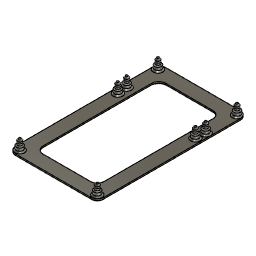
ESPBoardWithSenseHATHolder (Autodesk Fusion 360 design; units mm, degrees)
Autodesk Fusion 360 part; units mm, degrees
note: some values were not read from the file. Set by a fixed rule: which face or edge a step refers to.
sketch "Sketch1" plane through (0, 0, 0) normal (0, 0, 1) x (1, 0, 0)
  line L0 (27.5, -55) -> (-27.5, -55)
  line L1 (-32.5, -50) -> (-32.5, 50)
  line L2 (-27.5, 55) -> (27.5, 55)
  line L3 (32.5, 50) -> (32.5, -50)
  line L4 (32.5, -55) -> (-32.5, 55) construction
  line L5 (-32.5, -55) -> (32.5, 55) construction
  circle A0 centre (28.45, -51) radius 1.5
  circle A1 centre (28.45, 21) radius 1.5
  line L6 (28.45, -51) -> (28.45, 23.226) construction
  circle A2 centre (29, 28) radius 1.5
  line L7 (29, 28) -> (29, 54) construction
  circle A3 centre (29, 51) radius 1.5
  circle A4 centre (28.45, -51) radius 2.1
  circle A5 centre (28.45, 21) radius 2.1
  circle A6 centre (29, 28) radius 2.1
  circle A7 centre (29, 51) radius 2.1
  line L8 (29.3, 48.9) -> (28.7, 48.9)
  line L9 (28.7, 48.9) -> (28.7, 53.1)
  line L10 (28.7, 53.1) -> (29.3, 53.1)
  line L11 (29.3, 53.1) -> (29.3, 48.9)
  line L12 (29.3, 48.9) -> (28.7, 53.1) construction
  line L13 (28.7, 48.9) -> (29.3, 53.1) construction
  line L14 (29.3, 25.9) -> (28.7, 25.9)
  line L15 (28.7, 25.9) -> (28.7, 30.1)
  line L16 (28.7, 30.1) -> (29.3, 30.1)
  line L17 (29.3, 30.1) -> (29.3, 25.9)
  line L18 (29.3, 25.9) -> (28.7, 30.1) construction
  line L19 (28.7, 25.9) -> (29.3, 30.1) construction
  line L20 (28.75, 18.9) -> (28.15, 18.9)
  line L21 (28.15, 18.9) -> (28.15, 23.1)
  line L22 (28.15, 23.1) -> (28.75, 23.1)
  line L23 (28.75, 23.1) -> (28.75, 18.9)
  line L24 (28.75, 18.9) -> (28.15, 23.1) construction
  line L25 (28.15, 18.9) -> (28.75, 23.1) construction
  line L26 (28.75, -53.1) -> (28.15, -53.1)
  line L27 (28.15, -53.1) -> (28.15, -48.9)
  line L28 (28.15, -48.9) -> (28.75, -48.9)
  line L29 (28.75, -48.9) -> (28.75, -53.1)
  line L30 (28.75, -53.1) -> (28.15, -48.9) construction
  line L31 (28.15, -53.1) -> (28.75, -48.9) construction
  line L32 (0, 55) -> (0, -55) construction
  circle A8 centre (-29, 28) radius 2.1
  line L33 (-29.3, 30.1) -> (-29.3, 25.9)
  line L34 (-28.7, 48.9) -> (-28.7, 53.1)
  circle A9 centre (-28.45, 21) radius 2.1
  line L35 (-29.3, 48.9) -> (-28.7, 48.9)
  line L36 (-28.7, 48.9) -> (-29.3, 53.1) construction
  line L37 (-28.15, -53.1) -> (-28.75, -48.9) construction
  line L38 (-28.75, -53.1) -> (-28.15, -53.1)
  circle A10 centre (-28.45, 21) radius 1.5
  circle A11 centre (-28.45, -51) radius 1.5
  line L39 (-28.15, -53.1) -> (-28.15, -48.9)
  line L40 (-28.7, 25.9) -> (-29.3, 30.1) construction
  line L41 (-28.15, -48.9) -> (-28.75, -48.9)
  line L42 (-28.75, -48.9) -> (-28.75, -53.1)
  line L43 (-28.75, 18.9) -> (-28.15, 18.9)
  line L44 (-28.75, -53.1) -> (-28.15, -48.9) construction
  circle A12 centre (-28.45, -51) radius 2.1
  line L45 (-28.15, 18.9) -> (-28.75, 23.1) construction
  circle A13 centre (-29, 51) radius 2.1
  line L46 (-29.3, 53.1) -> (-29.3, 48.9)
  circle A14 centre (-29, 51) radius 1.5
  line L47 (-28.15, 18.9) -> (-28.15, 23.1)
  line L48 (-28.7, 30.1) -> (-29.3, 30.1)
  circle A15 centre (-29, 28) radius 1.5
  line L49 (-29.3, 25.9) -> (-28.7, 25.9)
  line L50 (-29.3, 48.9) -> (-28.7, 53.1) construction
  line L51 (-28.7, 25.9) -> (-28.7, 30.1)
  line L52 (-28.75, 23.1) -> (-28.75, 18.9)
  line L53 (-28.15, 23.1) -> (-28.75, 23.1)
  line L54 (-28.7, 53.1) -> (-29.3, 53.1)
  line L55 (-29.3, 25.9) -> (-28.7, 30.1) construction
  line L56 (-28.75, 18.9) -> (-28.15, 23.1) construction
  line L57 (17.5, -45) -> (-17.5, -45)
  line L58 (-22.5, -40) -> (-22.5, 40)
  line L59 (-17.5, 45) -> (17.5, 45)
  line L60 (22.5, 40) -> (22.5, -40)
  arc A16 (-17.5, 45) -> (-22.5, 40) centre (-17.5, 40) ccw
  arc A17 (-27.5, 55) -> (-32.5, 50) centre (-27.5, 50) ccw
  arc A18 (32.5, 50) -> (27.5, 55) centre (27.5, 50) ccw
  arc A19 (27.5, -55) -> (32.5, -50) centre (27.5, -50) ccw
  arc A20 (-32.5, -50) -> (-27.5, -55) centre (-27.5, -50) ccw
  arc A21 (-22.5, -40) -> (-17.5, -45) centre (-17.5, -40) ccw
  arc A22 (17.5, -45) -> (22.5, -40) centre (17.5, -40) ccw
  arc A23 (22.5, 40) -> (17.5, 45) centre (17.5, 40) ccw
  circle A24 centre (28.45, -51) radius 2.5
  circle A25 centre (28.45, 21) radius 2.5
  circle A26 centre (29, 28) radius 2.5
  circle A27 centre (29, 51) radius 2.5
  circle A28 centre (-29, 51) radius 2.5
  circle A29 centre (-29, 28) radius 2.5
  circle A30 centre (-28.45, 21) radius 2.5
  circle A31 centre (-28.45, -51) radius 2.5
  point P0 (29, 51)
  point P1 (29, 28)
  point P2 (28.45, 21)
  point P3 (28.45, -51)
  point P4 (-28.45, 23.226)
  point P5 (-28.45, 21)
  point P6 (-29, 28)
  point P7 (-29, 51)
  point P8 (-28.45, -51)
  point P9 (-28.45, -51)
  point P10 (-29, 28)
  dimension "d1" = 65
  dimension "d2" = 110
  dimension "d5" = 3
  dimension "d6" = 4.05
  dimension "d7" = 4
  dimension "d8" = 3
  dimension "d9" = 72
  dimension "d10" = 3
  dimension "d11" = 7
  dimension "d12" = 0.55
  dimension "d13" = 3
  dimension "d14" = 23
  dimension "d15" = 4.2
  dimension "d16" = 4.2
  dimension "d17" = 4.2
  dimension "d18" = 4.2
  dimension "d19" = 0.6
  dimension "d20" = 4.2
  dimension "d21" = 0.6
  dimension "d22" = 4.2
  dimension "d23" = 0.6
  dimension "d24" = 4.2
  dimension "d25" = 0.6
  dimension "d26" = 4.2
  dimension "d28" = 5
  dimension "d43" = 56.9
  dimension "d44" = 58
  dimension "d49" = 5
  dimension "d50" = 5
  dimension "d51" = 5
  dimension "d52" = 5
  constraint horizontal L0
  constraint perpendicular L0 L1
  constraint parallel L0 L2
  constraint parallel L1 L3
  constraint coincident L4 origin
  constraint coincident L5 origin
  constraint coincident P3 A0.centre
  constraint parallel L3 L6
  constraint coincident P2 L6
  constraint coincident P1 A2.centre
  constraint vertical L7
  constraint coincident L7 P0
  constraint concentric A0 A4
  constraint concentric A1 A5
  constraint concentric A2 A6
  constraint concentric A3 A7
  constraint horizontal L8
  constraint perpendicular L8 L9
  constraint parallel L8 L10
  constraint parallel L9 L11
  constraint coincident L12 P0
  constraint coincident L13 P0
  constraint coincident P0 A3.centre
  constraint horizontal L14
  constraint perpendicular L14 L15
  constraint parallel L14 L16
  constraint parallel L15 L17
  constraint coincident L18 P1
  constraint coincident L19 P1
  constraint horizontal L20
  constraint perpendicular L20 L21
  constraint parallel L20 L22
  constraint parallel L21 L23
  constraint coincident L24 P2
  constraint coincident L25 P2
  constraint coincident P2 A1.centre
  constraint horizontal L26
  constraint perpendicular L26 L27
  constraint parallel L26 L28
  constraint parallel L27 L29
  constraint coincident L30 P3
  constraint coincident L31 P3
  constraint symmetric A0 L32 A11
  constraint symmetric A1 L32 A10
  constraint symmetric P3 L32 P9
  constraint symmetric L6.end L32 P4
  constraint symmetric A2 L32 A15
  constraint symmetric P1 L32 P10
  constraint symmetric A3 L32 A14
  constraint symmetric A4 L32 A12
  constraint symmetric A5 L32 A9
  constraint symmetric A6 L32 A8
  constraint symmetric A7 L32 A13
  constraint symmetric L8.start L32 L35.start
  constraint symmetric L8.end L32 L34.start
  constraint symmetric L9.end L32 L34.end
  constraint symmetric L10.end L32 L36.end
  constraint symmetric P0 L32 P7
  constraint symmetric L14.start L32 L33.end
  constraint symmetric L14.end L32 L40.start
  constraint symmetric L15.end L32 L48.start
  constraint symmetric L16.end L32 L33.start
  constraint symmetric L20.start L32 L43.start
  constraint symmetric L20.end L32 L43.end
  constraint symmetric L21.end L32 L47.end
  constraint symmetric L22.end L32 L45.end
  constraint symmetric P2 L32 P5
  constraint symmetric L26.start L32 L38.start
  constraint symmetric L26.end L32 L37.start
  constraint symmetric L27.end L32 L39.end
  constraint symmetric L28.end L32 L37.end
  constraint tangent L58 A16
  constraint tangent L59 A16
  constraint coincident L2 L32.start
  constraint coincident L4.end L1
  constraint coincident L4.end L2
  constraint tangent L1 A17
  constraint tangent L2 A17
  constraint equal A16 A17
  constraint coincident L5.end L2
  constraint coincident L5.end L3
  constraint tangent L2 A18
  constraint tangent L3 A18
  constraint equal A16 A18
  constraint coincident L0 L32.end
  constraint coincident L4.start L3
  constraint coincident L4.start L0
  constraint tangent L3 A19
  constraint tangent L0 A19
  constraint equal A16 A19
  constraint coincident L5.start L0
  constraint coincident L5.start L1
  constraint tangent L0 A20
  constraint tangent L1 A20
  constraint equal A16 A20
  constraint tangent L57 A21
  constraint tangent L58 A21
  constraint equal A16 A21
  constraint tangent L60 A22
  constraint tangent L57 A22
  constraint equal A16 A22
  constraint tangent L60 A23
  constraint tangent L59 A23
  constraint equal A16 A23
  constraint concentric A5 A25
  constraint concentric A6 A26
  constraint concentric A7 A27
  constraint symmetric L32 A24 A31
  constraint symmetric L32 A25 A30
  constraint symmetric L32 A26 A29
  constraint symmetric L32 A27 A28
  measures "d1" distance of L4.end L5.end
  measures "d2" distance of L5.start L4.end
  measures "d5" diameter of A0
  measures "d6" distance of L3 P3
  measures "d7" distance of L0 P3
  measures "d8" diameter of A1
  measures "d9" vertical distance of P3 P2
  measures "d10" diameter of A2
  measures "d11" vertical distance of P2 P1
  measures "d12" distance of L6 P1
  measures "d13" diameter of A3
  measures "d14" distance of P1 P0
  measures "d15" diameter of A4
  measures "d16" diameter of A5
  measures "d17" diameter of A6
  measures "d18" diameter of A7
  measures "d19" distance of L9.end L10.end
  measures "d20" distance of L8.end L9.end
  measures "d21" distance of L15.end L16.end
  measures "d22" distance of L14.end L15.end
  measures "d23" distance of L21.end L22.end
  measures "d24" distance of L20.end L21.end
  measures "d25" distance of L27.end L28.end
  measures "d26" distance of L26.end L27.end
  measures "d28" radius of A16 L11
  measures "d43" distance of P3 P9
  measures "d44" distance of P0 P7
  measures "d49" diameter of A24
  measures "d50" diameter of A25
  measures "d51" diameter of A26
  measures "d52" diameter of A27
extrude "Extrude1" add sketch "Sketch1" against normal blind 2 contours L0 L1 L2 L3 A17 A18 A19 A20 | A0 L29 | A0 A4 L29 | A0 L27 L29 | A0 A4 L27 L29 | A0 A4 L27 L29 | A0 L27 | A0 A4 L27 | A4 L28 L29 | A4 L26 L29 | A4 L27 L28 | A4 L26 L27 | A1 L23 | A1 A5 L23 | A1 L21 L23 | A1 A5 L21 L23 | A1 A5 L21 L23 | A1 L21 | A1 A5 L21 | A5 L22 L23 | A5 L20 L23 | A5 L21 L22 | A5 L20 L21 | A2 L17 | A2 A6 L17 | A2 L15 L17 | A2 A6 L15 L17 | A2 A6 L15 L17 | A2 L15 | A2 A6 L15 | A6 L16 L17 | A6 L14 L17 | A6 L15 L16 | A6 L14 L15 | A3 L11 | A3 A7 L11 | A3 L9 L11 | A3 A7 L9 L11 | A3 A7 L9 L11 | A3 L9 | A3 A7 L9 | A7 L10 L11 | A7 L8 L11 | A7 L9 L10 | A7 L8 L9 | A8 A15 L51 | A8 L33 A15 L51 | A8 L48 L51 | A8 L49 L51 | A8 L33 A15 L51 | A8 L33 L48 | L33 A15 L51 | A15 L51 | A8 L33 L49 | A8 L33 A15 | L33 A15 | L34 L35 A13 | L34 A13 L46 A14 | L34 A13 A14 | L35 A13 L46 | L34 L46 A14 | L34 A14 | A13 L46 A14 | L34 A13 L46 A14 | L46 A14 | L34 A13 L54 | A13 L46 L54 | A9 A10 L47 | A9 A10 L47 L52 | A9 L47 L53 | A9 L43 L47 | A9 A10 L47 L52 | A9 L52 L53 | A10 L47 L52 | A10 L47 | A9 L43 L52 | A9 A10 L52 | A10 L52 | L38 L42 A12 | L38 L39 A12 | A11 L39 L42 A12 | A11 L42 A12 | A11 L39 A12 | A11 L39 L42 | A11 L42 | A11 L39 L42 A12 | L41 L42 A12 | A11 L39 | L39 L41 A12 | A24 | A25 | A26 | A27 | A28 | A29 | A30 | A31
extrude "Extrude2" add sketch "Sketch1" along normal blind 3 contours A0 L29 | A0 A4 L29 | A0 L27 L29 | A0 A4 L27 L29 | A0 A4 L27 L29 | A0 L27 | A0 A4 L27 | A4 L28 L29 | A4 L26 L29 | A4 L27 L28 | A4 L26 L27 | A1 L23 | A1 A5 L23 | A1 L21 L23 | A1 A5 L21 L23 | A1 A5 L21 L23 | A1 L21 | A1 A5 L21 | A5 L22 L23 | A5 L20 L23 | A5 L21 L22 | A5 L20 L21 | A2 L17 | A2 A6 L17 | A2 L15 L17 | A2 A6 L15 L17 | A2 A6 L15 L17 | A2 L15 | A2 A6 L15 | A6 L16 L17 | A6 L14 L17 | A6 L15 L16 | A6 L14 L15 | A3 L11 | A3 A7 L11 | A3 L9 L11 | A3 A7 L9 L11 | A3 A7 L9 L11 | A3 L9 | A3 A7 L9 | A7 L10 L11 | A7 L8 L11 | A7 L9 L10 | A7 L8 L9 | A8 A15 L51 | A8 L33 A15 L51 | A8 L48 L51 | A8 L49 L51 | A8 L33 A15 L51 | A8 L33 L48 | L33 A15 L51 | A15 L51 | A8 L33 L49 | A8 L33 A15 | L33 A15 | L34 L35 A13 | L34 A13 L46 A14 | L34 A13 A14 | L35 A13 L46 | L34 L46 A14 | L34 A14 | A13 L46 A14 | L34 A13 L46 A14 | L46 A14 | L34 A13 L54 | A13 L46 L54 | A9 A10 L47 | A9 A10 L47 L52 | A9 L47 L53 | A9 L43 L47 | A9 A10 L47 L52 | A9 L52 L53 | A10 L47 L52 | A10 L47 | A9 L43 L52 | A9 A10 L52 | A10 L52 | L38 L42 A12 | L38 L39 A12 | A11 L39 L42 A12 | A11 L42 A12 | A11 L39 A12 | A11 L39 L42 | A11 L42 | A11 L39 L42 A12 | L41 L42 A12 | A11 L39 | L39 L41 A12 | A24 | A25 | A26 | A27 | A28 | A29 | A30 | A31
extrude "Extrude3" add sketch "Sketch1" along normal blind 2.5 from surface at 3 contours A0 L29 | A0 L27 L29 | A0 L27 | A1 L23 | A1 L21 L23 | A1 L21 | A2 L17 | A2 L15 L17 | A2 L15 | A3 L11 | A3 L9 L11 | A3 L9 | L33 A15 L51 | A15 L51 | L33 A15 | L34 L46 A14 | L34 A14 | L46 A14 | A10 L47 L52 | A10 L47 | A10 L52 | A11 L39 L42 | A11 L42 | A11 L39
extrude "Extrude4" add sketch "Sketch1" along normal blind 2 draft -33 and the other way blind 0.5 draft -20 from surface at 5.5 contours A0 L29 | A0 A4 L29 | A0 L27 L29 | A0 A4 L27 L29 | A0 A4 L27 L29 | A0 L27 | A0 A4 L27 | A1 L23 | A1 A5 L23 | A1 L21 L23 | A1 A5 L21 L23 | A1 A5 L21 L23 | A1 L21 | A1 A5 L21 | A2 L17 | A2 A6 L17 | A2 L15 L17 | A2 A6 L15 L17 | A2 A6 L15 L17 | A2 L15 | A2 A6 L15 | A3 L11 | A3 A7 L11 | A3 L9 L11 | A3 A7 L9 L11 | A3 A7 L9 L11 | A3 L9 | A3 A7 L9 | A8 A15 L51 | A8 L33 A15 L51 | A8 L33 A15 L51 | L33 A15 L51 | A15 L51 | A8 L33 A15 | L33 A15 | L34 A13 L46 A14 | L34 A13 A14 | L34 L46 A14 | L34 A14 | A13 L46 A14 | L34 A13 L46 A14 | L46 A14 | A9 A10 L47 | A9 A10 L47 L52 | A9 A10 L47 L52 | A10 L47 L52 | A10 L47 | A9 A10 L52 | A10 L52 | A11 L39 L42 A12 | A11 L42 A12 | A11 L39 A12 | A11 L39 L42 | A11 L42 | A11 L39 L42 A12 | A11 L39
chamfer "Chamfer1" distance 1 angle 45 8 edges at (-30.7808, -50.096, 0) (26.1192, -50.096, 0) (26.1192, 21.904, 0) (26.6692, 28.904, 0) (-30.7808, 21.904, 0) (-31.3308, 28.904, 0) (-31.3308, 51.904, 0) (26.6692, 51.904, 0)
chamfer "Chamfer2" distance 1 angle 45 16 edges at (-31.0355, -53.5355, -2) (-32.5, 0, -2) (-31.0355, 53.5355, -2) (0, 55, -2) (31.0355, 53.5355, -2) (32.5, 0, -2) (31.0355, -53.5355, -2) (0, -55, -2) (0, -45, -2) (21.0355, -43.5355, -2) (22.5, 0, -2) (21.0355, 43.5355, -2) (0, 45, -2) (-21.0355, 43.5355, -2) (-22.5, 0, -2) (-21.0355, -43.5355, -2)
chamfer "Chamfer3" distance 1 distance2 0.6 8 edges at (27.0515, 21.5424, 3) (27.6015, 28.5424, 3) (27.6015, 51.5424, 3) (-30.3985, 51.5424, 3) (-30.3985, 28.5424, 3) (-29.8485, 21.5424, 3) (-29.8485, -50.4576, 3) (27.0515, -50.4576, 3) measured on face at (30.6018, 20.8013, 3) measured on face at (31.1518, 27.8013, 3) measured on face at (31.1518, 50.8013, 3) measured on face at (-26.8482, 50.8013, 3) measured on face at (-26.8482, 27.8013, 3) measured on face at (-26.2982, 20.8013, 3) measured on face at (-26.2926, -51.1242, 3) measured on face at (26.5975, -52.1127, 3)
fillet "Fillet1" radius 1 16 edges at (26.4921, 21.7594, 5.5) (26.6618, 20.3064, 5) (27.0421, 28.7594, 5.5) (27.2118, 27.3064, 5) (27.0421, 51.7594, 5.5) (27.2118, 50.3064, 5) (-30.9579, 51.7594, 5.5) (-30.7882, 50.3064, 5) (-30.9579, 28.7594, 5.5) (-30.7882, 27.3064, 5) (-30.4079, 21.7594, 5.5) (-30.2382, 20.3064, 5) (-30.4079, -50.2406, 5.5) (-30.2382, -51.6936, 5) (26.4921, -50.2406, 5.5) (26.6618, -51.6936, 5)
named bodies: "ESPBoardWithSenseHatHolder"
